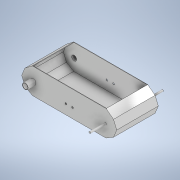
# Autodesk Inventor part: rama
Saved by Autodesk Inventor 2021 (Build 250183000, 183)
## iProperties
Created: 2021-06-23
Part Number: rama
Material: Generic
Document SubType Name: Modeling
Designer: Łukasz
Density: 1 g/cm^3
Appearance: Machined - Aluminum
Author: Łukasz
Autodesk Inventor part; units mm, degrees
ref_plane "YZ Plane" through (0, 0, 0) normal (1, 0, 0) x (0, 1, 0)
ref_plane "XZ Plane" through (0, 0, 0) normal (0, 1, 0) x (-1, 0, 0)
ref_plane "XY Plane" through (0, 0, 0) normal (0, 0, 1) x (1, 0, 0)
sketch "Sketch1" plane through (0, 0, 0) normal (0, 0, 1) x (1, 0, 0)
  circle A0 centre (0, 0) radius 11
  circle A1 centre (0, 0) radius 13
  dimension "d0" = 22
  dimension "d1" = 26
  constraints: 2 centre point, 2 coincident
  measures "d0" diameter of A0
  measures "d1" diameter of A1
extrude "Extrusion1" add sketch "Sketch1" along normal blind 35
sketch "Sketch3" plane through (0, 0, 35) normal (0, 0, 1) x (1, 0, 0)
  arc A0 (-11.1364, -38.4185) -> (-20.0192, 34.6299) centre (0, 0) ccw construction
  line L0 (0, 0) -> (0, -45) construction
  line L1 (0, 0) -> (-28.2843, -28.2843) construction
  line L2 (0, 0) -> (40, 0) construction
  line L3 (-40, 0) -> (-28.2843, -28.2843)
  line L4 (-28.2843, -28.2843) -> (0, -45)
  line L5 (-40, 0) -> (10, 0) construction
  line L6 (0, -45) -> (162.5, -45)
  line L7 (0, 50) -> (162.5, 50)
  line L8 (162.5, 0) -> (162.5, -45) construction
  line L9 (0, 0) -> (0, 50) construction
  line L10 (0, 0) -> (-28.2843, 28.2843) construction
  line L11 (0, 0) -> (40, 0) construction
  line L12 (-40, 0) -> (-28.2843, 28.2843)
  line L13 (-28.2843, 28.2843) -> (0, 50)
  line L14 (325, 0) -> (325, -45) construction
  line L15 (325, 0) -> (285, 0) construction
  line L16 (325, 0) -> (325, 50) construction
  line L17 (325, 0) -> (285, 0) construction
  circle A1 centre (325, 0) radius 14
  arc A2 (345.0192, 34.6299) -> (336.1364, -38.4185) centre (325, 0) ccw construction
  line L18 (353.2843, 28.2843) -> (325, 50)
  line L19 (353.2843, -28.2843) -> (325, -45)
  line L20 (325, 0) -> (353.2843, 28.2843) construction
  line L21 (325, 0) -> (353.2843, -28.2843) construction
  line L22 (365, 0) -> (353.2843, 28.2843)
  line L23 (365, 0) -> (353.2843, -28.2843)
  line L24 (365, 0) -> (315, 0) construction
  line L25 (325, -45) -> (162.5, -45)
  line L26 (325, 50) -> (162.5, 50)
  circle A3 centre (0, 0) radius 11 projected
  line L27 (162.5, 60) -> (-3.3961, 60)
  line L28 (-3.3961, 60) -> (-36.4982, 34.5853)
  line L29 (-36.4982, 34.5853) -> (-50.8239, 0)
  line L30 (-50.8239, 0) -> (-36.2457, -35.195)
  line L31 (-36.2457, -35.195) -> (-2.7341, -55)
  line L32 (-2.7341, -55) -> (162.5, -55)
  line L33 (162.5, -55) -> (327.7341, -55)
  line L34 (327.7341, -55) -> (361.2457, -35.195)
  line L35 (361.2457, -35.195) -> (375.8239, 0)
  line L36 (375.8239, 0) -> (361.4982, 34.5853)
  line L37 (361.4982, 34.5853) -> (328.3961, 60)
  line L38 (328.3961, 60) -> (162.5, 60)
  dimension "d14" = 80
  dimension "d15" = 45
  dimension "d16" = 135
  dimension "d17" = 162.5
  dimension "d18" = 135
  dimension "d19" = 50
  dimension "d42" = 10
  constraints: 78 end point, 12 symmetric about line, 5 horizontal, 5 point on line, 4 point on circle, 3 centre point, 2 coincident, 2 equal length, 2 perpendicular, 1 vertical, 12 other
  measures "d14" diameter of A0
  measures "d15" distance of L0.start L6.start
  measures "d16" angle of L1 L2
  measures "d17" distance of L6.start L6.end
  measures "d18" angle of L11 L10
  measures "d19" distance from line of point (0, 0) L7
  measures "d42" distance between parallel lines of L7 L27
extrude "Extrusion3" add sketch "Sketch3" along normal blind 2 contours L12 L13 L7 L26 L18 L22 L23 L19 L25 L6 L4 L3 | A1 | L38 L37 L36 L35 L34 L33 L32 L31 L30 L29 L28 L27
sketch "Sketch5" plane through (0, 0, 35) normal (0, 0, -1) x (-1, 0, 0)
  circle A0 centre (-325, 0) radius 4
  point P0 (0, 0)
  dimension "d22" = 8
  constraints: 2 coincident, 1 centre point
  measures "d22" diameter of A0
extrude "Extrusion4" add sketch "Sketch5" along normal blind 70
sketch "Sketch6" plane through (0, 0, 37) normal (0, 0, 1) x (1, 0, 0)
  line L0 (-28.2843, -28.2843) -> (0, -45) construction
  line L1 (0, -45) -> (325, -45) construction
  line L2 (325, -45) -> (353.2843, -28.2843) construction
  line L3 (353.2843, -28.2843) -> (365, 0) construction
  line L4 (365, 0) -> (353.2843, 28.2843) construction
  line L5 (353.2843, 28.2843) -> (325, 50) construction
  line L6 (325, 50) -> (0, 50) construction
  line L7 (0, 50) -> (-28.2843, 28.2843) construction
  line L8 (-28.2843, 28.2843) -> (-40, 0) construction
  line L9 (-40, 0) -> (-28.2843, -28.2843) construction
  circle A0 centre (0, 0) radius 11 projected
  line L10 (-3.3961, 60) -> (-36.4982, 34.5853) projected
  line L11 (-36.4982, 34.5853) -> (-50.8239, 0) projected
  line L12 (-50.8239, 0) -> (-36.2457, -35.195) projected
  line L13 (-36.2457, -35.195) -> (-2.7341, -55) projected
  line L14 (-2.7341, -55) -> (327.7341, -55) projected
  line L15 (327.7341, -55) -> (361.2457, -35.195) projected
  line L16 (361.2457, -35.195) -> (375.8239, 0) projected
  line L17 (375.8239, 0) -> (361.4982, 34.5853) projected
  line L18 (361.4982, 34.5853) -> (328.3961, 60) projected
  line L19 (328.3961, 60) -> (-3.3961, 60) projected
  line L20 (-2.7169, 58) -> (-34.8554, 33.3251)
  line L21 (-34.8554, 33.3251) -> (-48.6591, 0)
  line L22 (-48.6591, 0) -> (-34.6534, -33.8128)
  line L23 (-34.6534, -33.8128) -> (-2.1873, -53)
  line L24 (-2.1873, -53) -> (327.1873, -53)
  line L25 (327.1873, -53) -> (359.6534, -33.8128)
  line L26 (359.6534, -33.8128) -> (373.6591, 0)
  line L27 (373.6591, 0) -> (359.8554, 33.3251)
  line L28 (359.8554, 33.3251) -> (327.7169, 58)
  line L29 (-3.3961, 60) -> (-36.4982, 34.5853) projected
  line L30 (-3.3961, 60) -> (-3.3961, 57.4785)
  line L31 (328.3961, 60) -> (328.3961, 57.4785)
  line L32 (327.7169, 58) -> (314.5802, 58)
  line L33 (10.4198, 58) -> (-2.7169, 58)
  constraints: 26 end point, 4 point on line, 1 parallel, 1 perpendicular, 8 other
extrude "Extrusion5" add sketch "Sketch6" along normal blind 182.8 contours L30 L20 L21 L22 L23 L24 L25 L26 L27 L28 L31 L18 L17 L16 L15 L14 L13 L12 L11 L10
sketch "Sketch7" plane through (0, 0, 219.8) normal (0, 0, 1) x (1, 0, 0)
  line L0 (0, 50) -> (0, 47.4785) projected
  line L1 (0, 47.4785) -> (-26.6415, 27.0241) projected
  line L2 (-26.6415, 27.0241) -> (-37.8352, 0) projected
  line L3 (-37.8352, 0) -> (-26.692, -26.9021) projected
  line L4 (-26.692, -26.9021) -> (0.5468, -43) projected
  line L5 (0.5468, -43) -> (324.4532, -43) projected
  line L6 (324.4532, -43) -> (351.692, -26.9021) projected
  line L7 (351.692, -26.9021) -> (362.8352, 0) projected
  line L8 (362.8352, 0) -> (351.6415, 27.0241) projected
  line L9 (351.6415, 27.0241) -> (324.3208, 48) projected
  line L10 (324.3208, 48) -> (324.3208, 50) projected
  line L11 (325, 50) -> (324.3208, 50) projected
  line L12 (324.3208, 50) -> (324.3208, 48) projected
  line L13 (324.3208, 48) -> (351.6415, 27.0241) projected
  line L14 (351.6415, 27.0241) -> (362.8352, 0) projected
  line L15 (362.8352, 0) -> (351.692, -26.9021) projected
  line L16 (351.692, -26.9021) -> (324.4532, -43) projected
  line L17 (324.4532, -43) -> (0.5468, -43) projected
  line L18 (0.5468, -43) -> (-26.692, -26.9021) projected
  line L19 (-26.692, -26.9021) -> (-37.8352, 0) projected
  line L20 (-37.8352, 0) -> (-26.6415, 27.0241) projected
  line L21 (-26.6415, 27.0241) -> (0, 47.4785) projected
  line L22 (0, 47.4785) -> (0, 50) projected
  line L23 (0, 50) -> (-28.2843, 28.2843) projected
  line L24 (-28.2843, 28.2843) -> (-40, 0) projected
  line L25 (-40, 0) -> (-28.2843, -28.2843) projected
  line L26 (-28.2843, -28.2843) -> (0, -45) projected
  line L27 (0, -45) -> (325, -45) projected
  line L28 (325, -45) -> (353.2843, -28.2843) projected
  line L29 (353.2843, -28.2843) -> (365, 0) projected
  line L30 (365, 0) -> (353.2843, 28.2843) projected
  line L31 (353.2843, 28.2843) -> (325, 50) projected
  line L32 (325, 50) -> (353.2843, 28.2843) projected
  line L33 (353.2843, 28.2843) -> (365, 0) projected
  line L34 (365, 0) -> (353.2843, -28.2843) projected
  line L35 (353.2843, -28.2843) -> (325, -45) projected
  line L36 (325, -45) -> (0, -45) projected
  line L37 (0, -45) -> (-28.2843, -28.2843) projected
  line L38 (-28.2843, -28.2843) -> (-40, 0) projected
  line L39 (-40, 0) -> (-28.2843, 28.2843) projected
  line L40 (-28.2843, 28.2843) -> (0, 50) projected
  line L41 (324.3208, 50) -> (325, 50) projected
  circle A0 centre (0, 0) radius 11 projected
  line L42 (328.3961, 60) -> (328.3961, 57.4785) projected
  line L43 (328.3961, 57.4785) -> (359.8554, 33.3251) projected
  line L44 (359.8554, 33.3251) -> (373.6591, 0) projected
  line L45 (373.6591, 0) -> (359.6534, -33.8128) projected
  line L46 (359.6534, -33.8128) -> (327.1873, -53) projected
  line L47 (327.1873, -53) -> (-2.1873, -53) projected
  line L48 (-2.1873, -53) -> (-34.6534, -33.8128) projected
  line L49 (-34.6534, -33.8128) -> (-48.6591, 0) projected
  line L50 (-48.6591, 0) -> (-34.8554, 33.3251) projected
  line L51 (-34.8554, 33.3251) -> (-3.3961, 57.4785) projected
  line L52 (-3.3961, 57.4785) -> (-3.3961, 60) projected
  line L53 (-3.3961, 60) -> (-36.4982, 34.5853) projected
  line L54 (-36.4982, 34.5853) -> (-50.8239, 0) projected
  line L55 (-50.8239, 0) -> (-36.2457, -35.195) projected
  line L56 (-36.2457, -35.195) -> (-2.7341, -55) projected
  line L57 (-2.7341, -55) -> (327.7341, -55) projected
  line L58 (327.7341, -55) -> (361.2457, -35.195) projected
  line L59 (361.2457, -35.195) -> (375.8239, 0) projected
  line L60 (375.8239, 0) -> (361.4982, 34.5853) projected
  line L61 (361.4982, 34.5853) -> (328.3961, 60) projected
  line L62 (-3.3961, 60) -> (-3.3961, 57.4785) projected
  line L63 (-3.3961, 57.4785) -> (-34.8554, 33.3251) projected
  line L64 (-34.8554, 33.3251) -> (-48.6591, 0) projected
  line L65 (-48.6591, 0) -> (-34.6534, -33.8128) projected
  line L66 (-34.6534, -33.8128) -> (-2.1873, -53) projected
  line L67 (-2.1873, -53) -> (327.1873, -53) projected
  line L68 (327.1873, -53) -> (359.6534, -33.8128) projected
  line L69 (359.6534, -33.8128) -> (373.6591, 0) projected
  line L70 (373.6591, 0) -> (359.8554, 33.3251) projected
  line L71 (359.8554, 33.3251) -> (328.3961, 57.4785) projected
  line L72 (328.3961, 57.4785) -> (328.3961, 60) projected
  line L73 (328.3961, 60) -> (-3.3961, 60) projected
  circle A1 centre (0, 0) radius 11 projected
extrude "Extrusion6" add sketch "Sketch7" along normal blind 2 contours L0 L1 L2 L3 L4 L5 L6 L7 L8 L9 L10 L11 L31 L30 L29 L28 L27 L26 L25 L24 L23 | L61 L60 L59 L58 L57 L56 L55 L54 L53 L52 L51 L50 L49 L48 L47 L46 L45 L44 L43 L42 | L42 L43 L44 L45 L46 L47 L48 L49 L50 L51 L52 L73
sketch "Sketch8" plane through (0, 0, 221.8) normal (0, 0, 1) x (1, 0, 0)
  circle A0 centre (0, 0) radius 13 projected
  line L0 (0, 50) -> (-28.2843, 28.2843) projected
  line L1 (-28.2843, 28.2843) -> (-40, 0) projected
  line L2 (-40, 0) -> (-28.2843, -28.2843) projected
  line L3 (-28.2843, -28.2843) -> (0, -45) projected
  line L4 (0, -45) -> (325, -45) projected
  line L5 (325, -45) -> (353.2843, -28.2843) projected
  line L6 (353.2843, -28.2843) -> (365, 0) projected
  line L7 (365, 0) -> (353.2843, 28.2843) projected
  line L8 (353.2843, 28.2843) -> (325, 50) projected
  circle A1 centre (0, 0) radius 11 projected
  line L9 (324.3208, 50) -> (324.3208, 48) projected
  line L10 (324.3208, 48) -> (351.6415, 27.0241) projected
  line L11 (351.6415, 27.0241) -> (362.8352, 0) projected
  line L12 (362.8352, 0) -> (351.692, -26.9021) projected
  line L13 (351.692, -26.9021) -> (324.4532, -43) projected
  line L14 (324.4532, -43) -> (0.5468, -43) projected
  line L15 (0.5468, -43) -> (-26.692, -26.9021) projected
  line L16 (-26.692, -26.9021) -> (-37.8352, 0) projected
  line L17 (-37.8352, 0) -> (-26.6415, 27.0241) projected
  line L18 (-26.6415, 27.0241) -> (0, 47.4785) projected
  line L19 (0, 47.4785) -> (0, 50) projected
  line L20 (325, 50) -> (324.3208, 50) projected
extrude "Extrusion7" add sketch "Sketch8" along normal blind 35 contours A0
sketch "Sketch9" plane through (0, 0, 221.8) normal (0, 0, 1) x (1, 0, 0)
  circle A0 centre (325, 0) radius 4 projected
  point P0 (0, 0)
extrude "Extrusion8" add sketch "Sketch9" along normal blind 70
sketch "Sketch13" plane through (0, 0, 37) normal (0, 0, 1) x (1, 0, 0)
  circle A0 centre (147.5, -11.5574) radius 4 projected
  circle A1 centre (177.5, -11.5574) radius 4 projected
  point P0 (0, 0)
extrude "Extrusion12" cut sketch "Sketch13" against normal up to surface (2 mm away)
sketch "Sketch15" plane through (0, 0, 219.8) normal (0, 0, -1) x (-1, 0, 0)
  line L0 (0, 50) -> (28.2843, 28.2843) projected
  line L1 (28.2843, 28.2843) -> (40, 0) projected
  line L2 (40, 0) -> (28.2843, -28.2843) projected
  line L3 (28.2843, -28.2843) -> (0, -45) projected
  line L4 (0, -45) -> (-325, -45) projected
  line L5 (-325, -45) -> (-353.2843, -28.2843) projected
  line L6 (-353.2843, -28.2843) -> (-365, 0) projected
  line L7 (-365, 0) -> (-353.2843, 28.2843) projected
  line L8 (-353.2843, 28.2843) -> (-325, 50) projected
  line L9 (-324.3208, 50) -> (-324.3208, 48) projected
  line L10 (-324.3208, 48) -> (-351.6415, 27.0241) projected
  line L11 (-351.6415, 27.0241) -> (-362.8352, 0) projected
  line L12 (-362.8352, 0) -> (-351.692, -26.9021) projected
  line L13 (-351.692, -26.9021) -> (-324.4532, -43) projected
  line L14 (-324.4532, -43) -> (-0.5468, -43) projected
  line L15 (-0.5468, -43) -> (26.692, -26.9021) projected
  line L16 (26.692, -26.9021) -> (37.8352, 0) projected
  line L17 (37.8352, 0) -> (26.6415, 27.0241) projected
  line L18 (26.6415, 27.0241) -> (0, 47.4785) projected
  line L19 (0, 47.4785) -> (0, 50) projected
  line L20 (-325, 50) -> (-324.3208, 50) projected
  point P0 (0, 0)
sketch "Sketch16" plane through (0, 0, 219.8) normal (0, 0, -1) x (-1, 0, 0)
  circle A0 centre (-177.5, -11.5574) radius 4 projected
  circle A1 centre (-147.5, -11.5574) radius 4 projected
  point P0 (0, 0)
extrude "Extrusion13" cut sketch "Sketch16" against normal up to surface (2 mm away)
body "Solid1"
